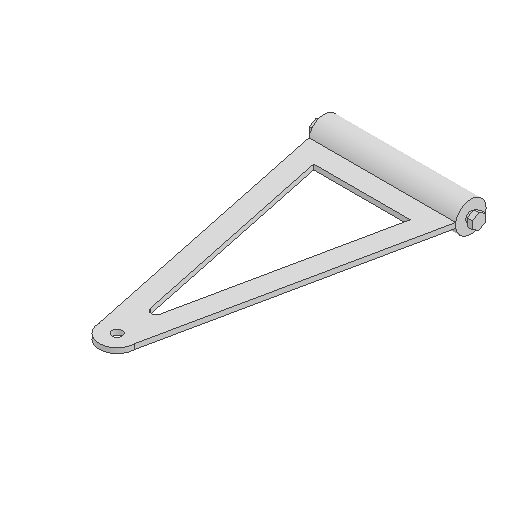
# Autodesk Inventor part: link
Saved by Autodesk Inventor 2025.2 (Build 292293000, 293)
## iProperties
Created: 2024-02-06
Part Number: link
Material: 일반
Document SubType Name: Modeling
Designer: ps737
Density: 1 g/cm^3
Appearance: 기본값
Author: ps737
Autodesk Inventor part; units mm, degrees
ref_plane "YZ Plane" through (0, 0, 0) normal (1, 0, 0) x (0, 1, 0)
ref_plane "XZ Plane" through (0, 0, 0) normal (0, 1, 0) x (-1, 0, 0)
ref_plane "XY Plane" through (0, 0, 0) normal (0, 0, 1) x (1, 0, 0)
sketch "스케치1" plane through (0, 0, 0) normal (1, 0, 0) x (0, 1, 0)
  circle A0 centre (0, 0) radius 15
  dimension "d0" = 30
  constraints: 1 centre point, 1 coincident
  measures "d0" diameter of A0
extrude "돌출1" add sketch "스케치1" along normal mid plane 144
sketch "스케치2" plane through (72, 0, 0) normal (1, 0, 0) x (0, 0, -1)
  circle A0 centre (0, 0) radius 5
  dimension "d3" = 10
  constraints: 1 centre point, 1 coincident
  measures "d3" diameter of A0
sketch "스케치3" plane through (-72, 0, 0) normal (-1, 0, 0) x (0, 0, 1)
  circle A0 centre (0, 0) radius 5
  dimension "d4" = 10
  constraints: 1 centre point, 1 coincident
  measures "d4" diameter of A0
extrude "돌출2" add sketch "스케치3" along normal blind 3
extrude "돌출3" add sketch "스케치2" along normal blind 3
sketch "스케치4" plane through (75, 0, 0) normal (1, 0, 0) x (0, 0, -1)
  line L0 (0, 7.5) -> (6.4952, 3.75)
  line L1 (6.4952, 3.75) -> (6.4952, -3.75)
  line L2 (6.4952, -3.75) -> (0, -7.5)
  line L3 (0, -7.5) -> (-6.4952, -3.75)
  line L4 (-6.4952, -3.75) -> (-6.4952, 3.75)
  line L5 (-6.4952, 3.75) -> (0, 7.5)
  point P0 (0, 0)
  point P1 (0, 0)
  dimension "d9" = 15
  constraints: 12 end point, 1 coincident, 13 other
  measures "d9" distance of L2.end L0.start
extrude "돌출4" add sketch "스케치4" along normal blind 5
sketch "스케치5" plane through (-75, 0, 0) normal (-1, 0, 0) x (0, 0, 1)
  circle A0 centre (0, 0) radius 5 projected
  line L0 (0, 7.5) -> (6.4952, 3.75)
  line L1 (6.4952, 3.75) -> (6.4952, -3.75)
  line L2 (6.4952, -3.75) -> (0, -7.5)
  line L3 (0, -7.5) -> (-6.4952, -3.75)
  line L4 (-6.4952, -3.75) -> (-6.4952, 3.75)
  line L5 (-6.4952, 3.75) -> (0, 7.5)
  dimension "d12" = 15
  constraints: 12 end point, 1 coincident, 13 other
  measures "d12" distance of L2.end L0.start
extrude "돌출5" add sketch "스케치5" along normal blind 5 contours A0 | L0 L1 L2 L3 L4 L5
sketch "스케치11" plane through (0, 0, 0) normal (0, 1, 0) x (-1, 0, 0)
  line L0 (72, 5) -> (72, -5) projected
  line L1 (72, 0) -> (72, 275)
  line L2 (-72, 15) -> (-72, -15) projected
  line L3 (72, 275) -> (-72, 275)
  line L4 (-72, 275) -> (-72, 0)
  line L5 (72, 0) -> (-72, 0)
  line L6 (-75, 6.4952) -> (-75, 0) projected
  point P0 (0, 0)
  dimension "d32" = 275
  constraints: 8 end point, 2 midpoint, 1 horizontal, 1 perpendicular, 1 vertical
  measures "d32" distance of L1.start L1.end
extrude "돌출12" add sketch "스케치11" along normal mid plane 5
sketch "스케치12" plane through (0, 2.5, 0) normal (0, 1, 0) x (1, 0, 0)
  line L0 (-72, -14.7902) -> (72, -14.7902) projected
  line L1 (-72, -14.7902) -> (-17.5, -275)
  line L2 (-72, -275) -> (72, -275) projected
  line L3 (0, -275) -> (0, -66.6038)
  line L4 (72, -14.7902) -> (17.5, -275)
  line L5 (-72, -14.7902) -> (-72, -275) projected
  line L6 (72, -275) -> (72, -14.7902) projected
  point P0 (0, 0)
  dimension "d37" = 35
  constraints: 6 end point, 1 point on line, 1 symmetric about line, 1 vertical
  measures "d37" distance of L4.end L1.end
extrude "돌출13" cut sketch "스케치12" against normal blind 5 contours L1 L2 L5 | L6 L2 L4
sketch "스케치13" plane through (0, 2.5, 0) normal (0, 1, 0) x (1, 0, 0)
  line L0 (-17.5, -275) -> (17.5, -275) projected
  circle A0 centre (0, -275) radius 17.5
  point P0 (0, 0)
  constraints: 1 midpoint, 3 other
extrude "돌출14" add sketch "스케치13" against normal blind 5 contours L0 A0 picked at (2.0685, -280.4543)
sketch "스케치14" plane through (0, 2.5, 0) normal (0, 1, 0) x (1, 0, 0)
  arc A0 (-17.5, -275) -> (17.5, -275) centre (0, -275) ccw projected
  circle A1 centre (0, -275) radius 5
  line L0 (-72, -14.7902) -> (-17.5, -275) projected
  line L1 (17.5, -275) -> (72, -14.7902) projected
  line L2 (-72, -14.7902) -> (72, -14.7902) projected
  line L3 (-72, -14.7902) -> (-17.5, -275) projected
  arc A2 (-17.5, -275) -> (17.5, -275) centre (0, -275) ccw projected
  line L4 (47.3771, -34.7902) -> (4.8938, -237.6263)
  line L5 (-4.8938, -237.6263) -> (-47.3771, -34.7902)
  line L6 (-47.3771, -34.7902) -> (47.3771, -34.7902)
  arc A3 (-4.8938, -237.6263) -> (4.8938, -237.6263) centre (0, -236.6013) ccw
  point P0 (0, 0)
  dimension "d40" = 10
  dimension "d41" = 20
  dimension "d42" = 5
  constraints: 6 end point, 2 centre point, 2 point on circle, 2 tangent, 1 coincident, 2 other
  measures "d40" diameter of A1
  measures "d41" distance between parallel lines of L1 L4
  measures "d42" radius of A3
extrude "돌출15" cut sketch "스케치14" against normal blind 5 contours A1 | L4 A3 L5 L6
